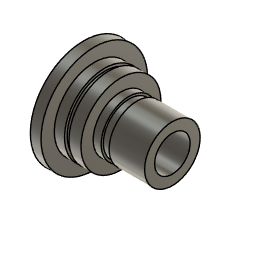
Turning Video Tutorial (Autodesk Fusion 360 design; units mm, degrees)
Autodesk Fusion 360 part; units mm, degrees
sketch "Sketch1" plane through (0, 0, 0) normal (0, 1, 0) x (1, 0, 0)
  line L0 (0, 0) -> (0, -30.48)
  line L1 (0, 0) -> (50.8, 0)
  line L2 (50.8, 0) -> (50.8, -15.875)
  line L3 (50.8, -15.875) -> (30.48, -15.875)
  line L4 (30.48, -15.875) -> (30.48, -14.6152)
  line L5 (30.48, -14.6152) -> (25.908, -14.6152)
  line L6 (25.908, -14.6152) -> (25.908, -15.875)
  line L7 (25.908, -15.875) -> (21.336, -15.875)
  line L8 (21.336, -15.875) -> (21.336, -22.86)
  line L9 (21.336, -22.86) -> (14.478, -22.86)
  line L10 (14.478, -22.86) -> (14.478, -21.336)
  line L11 (14.478, -21.336) -> (11.938, -21.336)
  line L12 (11.938, -21.336) -> (11.938, -22.86)
  line L13 (11.938, -22.86) -> (6.096, -22.86)
  line L14 (6.096, -22.86) -> (6.096, -30.48)
  line L15 (6.096, -30.48) -> (0, -30.48)
  line L16 (50.8, -10.16) -> (0, -10.16)
  dimension "d1" = 30.48
  dimension "d2" = 50.8
  dimension "d3" = 15.875
  dimension "d4" = 20.32
  dimension "d5" = 2.54
  dimension "d6" = 29.464
  dimension "d7" = 36.322
  dimension "d8" = 22.86
  dimension "d9" = 44.704
  dimension "d10" = 1.524
  dimension "d11" = 14.6152
  dimension "d12" = 10.16
  constraint coincident L0.start L1.start
  constraint vertical L0
  constraint perpendicular L0 L1
  constraint perpendicular L1 L2
  constraint perpendicular L2 L3
  constraint perpendicular L3 L4
  constraint perpendicular L4 L5
  constraint perpendicular L5 L6
  constraint perpendicular L6 L7
  constraint perpendicular L7 L8
  constraint perpendicular L8 L9
  constraint perpendicular L9 L10
  constraint perpendicular L10 L11
  constraint perpendicular L11 L12
  constraint perpendicular L12 L13
  constraint perpendicular L13 L14
  constraint collinear L9 L13
  constraint collinear L3 L7
  constraint horizontal L15
  constraint equal L5 L7
  constraint perpendicular L0 L16
  constraint coincident L0 L16.end
  constraint coincident L2 L16.start
  measures "d1" distance of L0.start L0.end
  measures "d2" distance of L0.start L1.end
  measures "d3" distance of L1.end L2.end
  measures "d4" distance of L2.end L3.end
  measures "d5" distance of L10.end L11.end
  measures "d6" distance of L2 L8
  measures "d7" distance of L2 L10
  measures "d8" distance of L1 L13
  measures "d9" distance of L2 L14
  measures "d10" distance of L11 L13
  measures "d11" distance of L1 L5
  measures "d12" distance of L1 L16
revolve "Revolve1" add sketch "Sketch1" angle 360 about axis through (0, 0, 0) along (1, 0, 0) contours L0 L2 L3 L4 L5 L6 L7 L8 L9 L10 L11 L12 L13 L14 L15 L16
equation "d11 = ( 1.1508 / 2 ) * 1 in"
